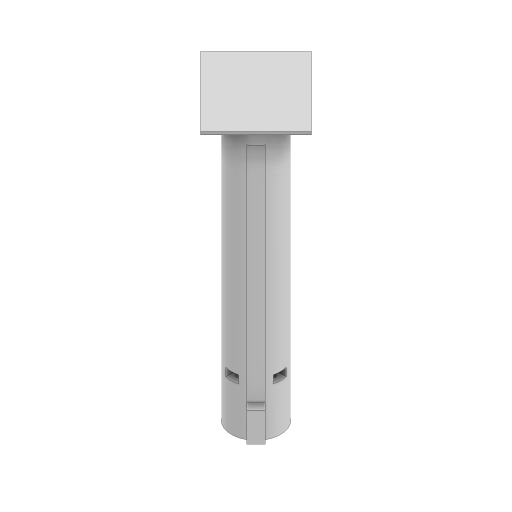
# Autodesk Inventor part: PART_5_1
Saved by Autodesk Inventor 2024 (Build 280153000, 153)
## iProperties
Created: 2024-08-20
Part Number: PART_5_1
Material: Generic
Document SubType Name: Modeling
Designer: Jhuliams
Density: 1 g/cm^3
Appearance: Default
Author: Jhuliams
Autodesk Inventor part; units mm, degrees
ref_plane "YZ Plane" through (0, 0, 0) normal (1, 0, 0) x (0, 1, 0)
ref_plane "XZ Plane" through (0, 0, 0) normal (0, 1, 0) x (-1, 0, 0)
ref_plane "XY Plane" through (0, 0, 0) normal (0, 0, 1) x (1, 0, 0)
sketch "Sketch11" plane through (0, 0, 0) normal (0, 1, 0) x (-1, 0, 0)
  circle A0 centre (0, 0) radius 12.5
  dimension "d32" = 25
  constraints: 1 centre point, 1 coincident
  measures "d32" diameter of A0
extrude "Extrusion10" add sketch "Sketch11" along normal blind 140
sketch "Sketch12" plane through (0, 0, 0) normal (0, -1, 0) x (1, 0, 0)
  circle A0 centre (0, 0) radius 5.25
  dimension "d35" = 10.5
  constraints: 1 centre point, 1 coincident
  measures "d35" diameter of A0
extrude "Extrusion11" cut sketch "Sketch12" against normal blind 10.3
sketch "Sketch13" plane through (0, 0, 0) normal (0, -1, 0) x (1, 0, 0)
  circle A0 centre (0, 0) radius 11.15
  dimension "d38" = 22.3
  constraints: 1 centre point, 1 coincident
  measures "d38" diameter of A0
extrude "Extrusion12" cut sketch "Sketch13" against normal blind 3.8
sketch "Sketch14" plane through (0, 3.8, 0) normal (0, -1, 0) x (1, 0, 0)
  circle A0 centre (0, 0) radius 8
  circle A1 centre (0, -8) radius 1.75
  circle A2 centre (8, 0) radius 1.75
  circle A3 centre (0, 8) radius 1.75
  circle A4 centre (-8, 0) radius 1.75
  dimension "d41" = 16
  dimension "d42" = 3.5
  dimension "d45" = 360
  constraints: 4 centre point, 1 coincident, 1 vertical alignment, 11 other
  measures "d42" diameter of A1
extrude "Extrusion13" cut sketch "Sketch14" against normal blind 30 contours A0 A2 | A0 A2 | A3 A0 | A0 A3 | A1 A0 | A0 A1 | A4 A0 | A0 A4
ref_plane "Work Plane1" through (0, 18.8, 0) normal (0, -1, 0) x (1, 0, 0)
sketch "Sketch15" plane through (0, 18.8, 0) normal (0, -1, 0) x (1, 0, 0)
  circle A0 centre (8, 0) radius 1.75 projected
  circle A1 centre (8, 0) radius 1.75 projected
  circle A2 centre (0, 8) radius 1.75 projected
  circle A3 centre (0, 8) radius 1.75 projected
  circle A4 centre (0, -8) radius 1.75 projected
  circle A5 centre (0, -8) radius 1.75 projected
  circle A6 centre (-8, 0) radius 1.75 projected
  circle A7 centre (-8, 0) radius 1.75 projected
  line L0 (8, 0) -> (8, -3.2)
  line L1 (8, -3.2) -> (5.2287, -1.6)
  line L2 (5.2287, -1.6) -> (5.2287, 1.6)
  line L3 (5.2287, 1.6) -> (8, 3.2)
  line L4 (8, 3.2) -> (10.7713, 1.6)
  line L5 (10.7713, 1.6) -> (10.7713, -1.6)
  line L6 (10.7713, -1.6) -> (8, -3.2)
  line L7 (8, 3.2) -> (13.6081, 3.2)
  line L8 (13.6081, 3.2) -> (13.6081, -3.2)
  line L9 (13.6081, -3.2) -> (8, -3.2)
  circle A8 centre (0, 0) radius 8
  line L10 (1.6, 5.2287) -> (-1.6, 5.2287)
  line L11 (-1.6, 5.2287) -> (-3.2, 8)
  line L12 (3.2, 8) -> (1.6, 5.2287)
  line L13 (-3.2, 8) -> (-1.6, 10.7713)
  line L14 (-1.6, 10.7713) -> (1.6, 10.7713)
  line L15 (1.6, 10.7713) -> (3.2, 8)
  line L16 (-3.2, 8) -> (-3.2, 13.6081)
  line L17 (-3.2, 13.6081) -> (3.2, 13.6081)
  line L18 (3.2, 13.6081) -> (3.2, 8)
  line L19 (-5.2287, 1.6) -> (-5.2287, -1.6)
  line L20 (-5.2287, -1.6) -> (-8, -3.2)
  line L21 (-8, 3.2) -> (-5.2287, 1.6)
  line L22 (-8, -3.2) -> (-10.7713, -1.6)
  line L23 (-10.7713, -1.6) -> (-10.7713, 1.6)
  line L24 (-10.7713, 1.6) -> (-8, 3.2)
  line L25 (-8, -3.2) -> (-13.6081, -3.2)
  line L26 (-13.6081, -3.2) -> (-13.6081, 3.2)
  line L27 (-13.6081, 3.2) -> (-8, 3.2)
  line L28 (-1.6, -5.2287) -> (1.6, -5.2287)
  line L29 (1.6, -5.2287) -> (3.2, -8)
  line L30 (-3.2, -8) -> (-1.6, -5.2287)
  line L31 (3.2, -8) -> (1.6, -10.7713)
  line L32 (1.6, -10.7713) -> (-1.6, -10.7713)
  line L33 (-1.6, -10.7713) -> (-3.2, -8)
  line L34 (3.2, -8) -> (3.2, -13.6081)
  line L35 (3.2, -13.6081) -> (-3.2, -13.6081)
  line L36 (-3.2, -13.6081) -> (-3.2, -8)
  dimension "d50" = 3.2
  dimension "d51" = 16
  dimension "d54" = 360
  constraints: 74 end point, 2 coincident, 2 perpendicular, 1 centre point, 1 horizontal, 1 vertical, 82 other
  measures "d50" distance of L0.start L0.end
  measures "d51" diameter of A8
extrude "Extrusion14" cut sketch "Sketch15" against normal blind 4 contours A0 A8 L3 L4 L5 L6 L0 | A0 A8 L1 L2 L3 | L0 L1 A8 A0 | L6 L5 L4 L7 L8 L9 | L12 L10 L11 A8 A2 | A8 A2 L11 L13 L14 L15 L12 | L29 L31 L32 L33 L30 A8 A4 | A8 A4 L30 L28 L29 | L15 L14 L13 L16 L17 L18 | L34 L35 L36 L33 L32 L31 | L21 L19 L20 A8 A6 | A8 A6 L20 L22 L23 L24 L21 | L24 L23 L22 L25 L26 L27
sketch "Sketch16" plane through (0, 10.3, 0) normal (0, -1, 0) x (1, 0, 0)
  circle A0 centre (0, 0) radius 4.15
  dimension "d61" = 8.3
  constraints: 1 centre point, 1 coincident
  measures "d61" diameter of A0
extrude "Extrusion15" cut sketch "Sketch16" against normal blind 126
sketch "Sketch18" plane through (0, 0, 0) normal (0, -1, 0) x (1, 0, 0)
  line L0 (0, 0) -> (8.8388, 8.8388)
  circle A0 centre (0, 0) radius 12.5 projected
  line L1 (0, 0) -> (12.5, 0) construction
  line L2 (8.8388, 8.8388) -> (10.4652, 10.4652)
  line L3 (12.7633, 8.1671) -> (11.1369, 6.5407)
  line L4 (11.1369, 6.5407) -> (7.8462, 3.25)
  line L5 (7.8462, 3.25) -> (12.5, 3.25)
  line L6 (8.1671, 12.7633) -> (6.5407, 11.1369)
  line L7 (6.5407, 11.1369) -> (-7.8462, -3.25)
  line L8 (-7.8462, -3.25) -> (12.5, -3.25)
  line L9 (8.1671, 12.7633) -> (12.7633, 8.1671)
  line L10 (5.869, 10.4652) -> (10.4652, 5.869)
  point P0 (6.2368, 10.833)
  point P1 (10.833, 6.2368)
  dimension "d64" = 45
  dimension "d65" = 2.3
  dimension "d66" = 3.25
  dimension "d67" = 3.25
  constraints: 22 end point, 2 point on line, 1 equal length, 1 horizontal, 1 perpendicular, 6 other
  measures "d64" angle of L1 L0
  measures "d65" distance of L0.end L2.end
  measures "d66" distance between parallel lines of L2 L3
  measures "d67" distance between parallel lines of L0 L7
extrude "Extrusion16" add sketch "Sketch18" against normal blind 10 contours L2 L9 L3 L4 A0 | A0 L7 L6 L9 L2
sketch "Sketch20" plane through (0, 140, 0) normal (0, 1, 0) x (1, 0, 0)
  line L0 (3.5355, -31.8198) -> (-31.8198, 3.5355)
  line L1 (-31.8198, 3.5355) -> (-3.5355, 31.8198)
  line L2 (-3.5355, 31.8198) -> (31.8198, -3.5355)
  line L3 (31.8198, -3.5355) -> (3.5355, -31.8198)
  line L4 (3.5355, -31.8198) -> (-3.5355, 31.8198) construction
  line L5 (-31.8198, 3.5355) -> (31.8198, -3.5355) construction
  point P0 (0, 0)
  dimension "d75" = 50
  dimension "d76" = 40
  constraints: 12 end point, 2 parallel, 1 perpendicular
  measures "d75" distance of L1.end L2.end
  measures "d76" distance of L0.end L1.end
extrude "Extrusion18" add sketch "Sketch20" against normal blind 5
fillet "Fillet3" radius 2 1 edges at (12.5, 135, 0)
sketch "Sketch21" plane through (12.7633, 0, 8.1671) normal (0.7071068, 0, 0.7071068) x (0.7071068, 0, -0.7071068)
  line L0 (-6.5, 10) -> (0, 10)
  line L1 (0, 10) -> (0, 125)
  line L2 (0, 125) -> (-6.5, 125)
  line L3 (-6.5, 125) -> (-6.5, 10)
  point P0 (-3.25, 0)
  dimension "d80" = 6.5
  dimension "d81" = 115
  constraints: 8 end point, 2 parallel, 1 horizontal, 1 perpendicular
  measures "d80" distance of L2.end L1.end
  measures "d81" distance of L1.end L0.end
extrude "Extrusion19" cut sketch "Sketch21" against normal blind 5
sketch "Sketch22" plane through (0, 0, 0) normal (0, -1, 0) x (1, 0, 0)
  circle A0 centre (0, 0) radius 11.15 projected
  arc A1 (6.2368, 10.833) -> (10.833, 6.2368) centre (0, 0) ccw projected
  line L0 (10.833, 6.2368) -> (12.7633, 8.1671) projected
  line L1 (12.7633, 8.1671) -> (8.1671, 12.7633) projected
  line L2 (8.1671, 12.7633) -> (6.2368, 10.833) projected
extrude "Extrusion20" add sketch "Sketch22" along normal blind 5
chamfer "Chamfer4" distance 5 angle 45 1 edges at (17.6777, 135, 17.6777)
body "Solid3"
